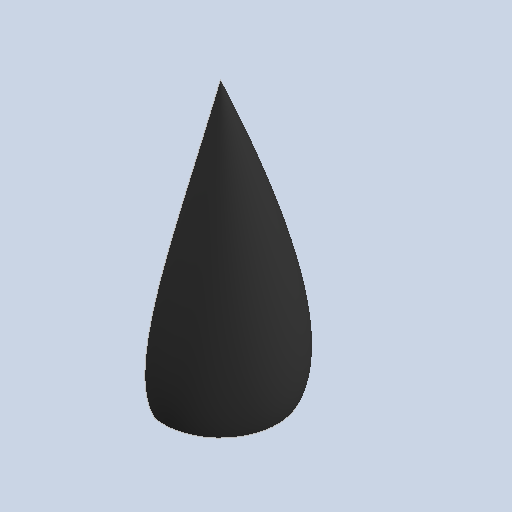
# Autodesk Inventor part: newleg
Saved by Autodesk Inventor 2023 (Build 270158000, 158)
## iProperties
Created: 2022-11-17
Part Number: newleg
Material: ゴム、黒
Document SubType Name: Modeling
Designer: 野口　裕太
Density: 0.93 g/cm^3
Appearance: ゴム - 黒
Author: 野口　裕太
Autodesk Inventor part; units mm, degrees
ref_plane "YZ Plane" through (0, 0, 0) normal (1, 0, 0) x (0, 1, 0)
ref_plane "XZ Plane" through (0, 0, 0) normal (0, 1, 0) x (-1, 0, 0)
ref_plane "XY Plane" through (0, 0, 0) normal (0, 0, 1) x (1, 0, 0)
sketch "スケッチ1" plane through (0, 0, 0) normal (0, 0, 1) x (1, 0, 0)
  line L0 (0, 0) -> (0, 40)
  line L1 (0, 40) -> (0, 190)
  line L2 (0, 40) -> (-45, 40)
  line L3 (0, 0) -> (-40, 0)
  spline S0 degree 2 poles (-40, 0) (-61.343, 41.3687) (0, 190) knots 0 0 0 1 1 1
  point P0 (0, 100)
  dimension "d0" = 40
  dimension "d1" = 150
  dimension "d2" = 45
  dimension "d3" = 40
  dimension "d14" = 100
  constraints: 8 end point, 2 horizontal, 2 point on line, 1 vertical, 3 other
  measures "d0" distance of L0.start L0.end
  measures "d1" distance of L0.end L1.end
  measures "d2" distance of L0.end L2.end
  measures "d3" distance of L0.start L3.end
  measures "d14" distance from line of L3 point (0, 100)
revolve "回転1" add sketch "スケッチ1" angle 360 about axis through (0, 40, 0) along (0, 1, 0)
sketch "スケッチ4" plane through (0, 0, 0) normal (0, -1, 0) x (1, 0, 0)
  circle A0 centre (0, 0) radius 40 projected
  line L0 (-30, -26.4575) -> (-30, 26.4575)
  circle A1 centre (0, 0) radius 50.9747
  line L1 (-30, -41.2119) -> (-30, 41.2119)
  point P0 (-30, 0)
  point P1 (-40, 0)
  dimension "d15" = 30
  constraints: 4 end point, 4 point on circle, 1 centre point, 1 coincident, 1 point on line, 1 vertical
  measures "d15" distance of point (0, 0) point (-30, 0)
extrude "押し出し3" cut sketch "スケッチ4" against normal blind 400 contours L0 A0 | A0 L1 A1 picked at (-33.2623, -1.3742) picked at (-32.3949, 34.1789)
sketch "スケッチ5" plane through (-30, 0, -26.4575) normal (-1, 0, 0) x (0, 0, 1)
  line L0 (52.915, 0) -> (0, 0) projected
  point P0 (26.4575, 0)
  point P1 (26.4575, 0)
  point P2 (16.4575, 100)
  point P3 (16.4575, 130)
  point P4 (36.4575, 100)
  point P5 (36.4575, 130)
  dimension "d20" = 30
  constraints: 1 midpoint
  measures "d20" distance of point (16.458, 100) point (16.458, 130)
hole "穴1" at (-30, 100, -10) at (-30, 130, -10) at (-30, 130, 10) at (-30, 100, 10) direction (1, 0, 0) diameter 2.6 depth 40
sketch "スケッチ6" plane through (0, 0, 0) normal (0, -1, 0) x (1, 0, 0)
  circle A0 centre (-125, 0) radius 125
  point P0 (0, 0)
  dimension "d28" = 250
  dimension "d29" = 125
  constraints: 1 centre point
  measures "d28" diameter of A0
  measures "d29" distance of point (0, 0) A0.centre
extrude "押し出し4" cut sketch "スケッチ6" against normal blind 400
sketch "スケッチ7" plane through (0, 0, 0) normal (0, -1, 0) x (1, 0, 0)
  circle A0 centre (0, 0) radius 32.5
  dimension "d32" = 65
  constraints: 1 centre point, 1 coincident
  measures "d32" diameter of A0
extrude "押し出し5" cut sketch "スケッチ7" against normal blind 70
fillet "フィレット2" radius 7 1 edges at (32.5, 70, 0)
